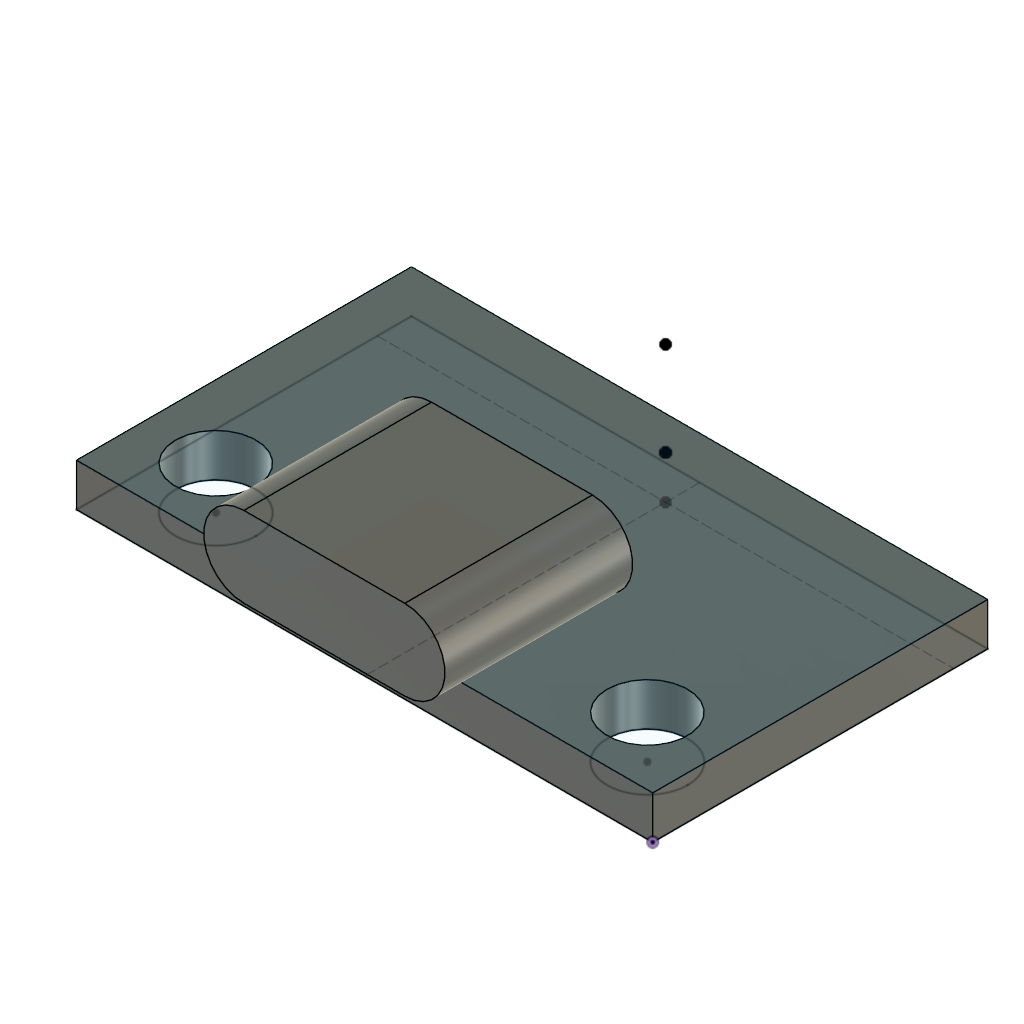
USB-Breakout (Autodesk Fusion 360 design; units mm, degrees)
Autodesk Fusion 360 part; units mm, degrees
sketch "Skizze1" plane through (0, 0, 0) normal (0, 0, 1) x (1, 0, 0)
  line L0 (0, 0) -> (-21.5, 0)
  line L1 (-21.5, 0) -> (-21.5, 12.5)
  line L2 (-21.5, 12.5) -> (0, 12.5)
  line L3 (0, 12.5) -> (0, 0)
  circle A0 centre (-18.8, 2.5) radius 1.5
  circle A1 centre (-2.7, 2.5) radius 1.5
  line L4 (-21.5, 11.23) -> (0, 11.23) construction
  line L5 (-10.75, 12.5) -> (-10.75, 0) construction
  point P0 (-10.75, 11.23)
  dimension "d1" = 21.5
  dimension "d2" = 12.5
  dimension "d3" = 3
  dimension "d4" = 2.7
  dimension "d5" = 2.7
  dimension "d6" = 2.5
  dimension "d7" = 2.5
  dimension "d8" = 1.27
  constraint horizontal L0
  constraint vertical L1
  constraint horizontal L2
  constraint vertical L3
  constraint coincident L0.start L3.end
  constraint equal A0 A1
  constraint coincident L1 L4.start
  constraint coincident L3 L4.end
  constraint perpendicular L3 L4
  constraint midpoint L2 L5.start
  constraint midpoint L0 L5.end
  constraint midpoint L4 P0
  measures "d1" distance of L1.end L2.end
  measures "d2" distance of L0.end L1.end
  measures "d3" diameter of A0
  measures "d4" distance of L1 A0.centre
  measures "d5" distance of L3 A1.centre
  measures "d6" distance of L0 A0.centre
  measures "d7" distance of L0 A1.centre
  measures "d8" distance of L2 L4
extrude "Extrusion1" add sketch "Skizze1" along normal blind 1.6
sketch "Skizze2" plane through (0, 0, 0) normal (0, -1, 0) x (1, 0, 0)
  line L0 (-21.5, 0) -> (0, 0)
  line L1 (0, 0) -> (0, 1.6)
  line L2 (0, 1.6) -> (-21.5, 1.6)
  line L3 (-21.5, 1.6) -> (-21.5, 0)
  line L4 (-10.75, 0) -> (-10.75, 13.6465) construction
  line L5 (-13.75, 4.6) -> (-7.75, 4.6)
  line L6 (-7.75, 1.6) -> (-13.75, 1.6)
  arc A0 (-13.75, 4.6) -> (-13.75, 1.6) centre (-13.75, 3.1) ccw
  arc A1 (-7.75, 1.6) -> (-7.75, 4.6) centre (-7.75, 3.1) ccw
  point P0 (-10.75, 1.6)
  dimension "d11" = 1.5
  dimension "d12" = 6
  constraint midpoint L0 L4.start
  constraint perpendicular L2 L4
  constraint tangent L5 A1
  constraint tangent L6 A0
  constraint tangent L5 A0
  constraint tangent L6 A1
  constraint equal A0 A1
  constraint symmetric L4 L5.start L5.end
  constraint midpoint L2 P0
  constraint coincident L6 P0
  measures "d11" radius of A0
  measures "d12" distance of A0.centre A1.centre
extrude "Extrusion2" add sketch "Skizze2" along normal blind 1.5 and the other way blind 5.5 contours L2 L5 L6 A0 A1
sketch "Skizze3" plane through (0, 0, 1.6) normal (0, 0, 1) x (-1, 0, 0)
  line L0 (7.75, -5.5) -> (7.75, 0)
  line L1 (7.75, 0) -> (0, 0)
  line L2 (0, 0) -> (0, -12.5)
  line L3 (0, -12.5) -> (21.5, -12.5)
  line L4 (21.5, -12.5) -> (21.5, 0)
  line L5 (21.5, 0) -> (13.75, 0)
  line L6 (13.75, 0) -> (13.75, -5.5)
  line L7 (13.75, -5.5) -> (7.75, -5.5)
  circle A0 centre (2.7, -2.5) radius 1.5
  circle A1 centre (18.8, -2.5) radius 1.5
  point P0 (10.75, -11.23)
  point P1 (10.75, -11.23)
  constraint coincident P1 P0
ref_plane "Arbeitsebene1" through (0, 0, 5.1) normal (0, 0, 1) x (1, 0, 0)
sketch "Skizze4" plane through (0, 0, 5.1) normal (0, 0, 1) x (1, 0, 0)
  point P0 (-10.75, 11.23)
  point P1 (-10.75, 11.23)
  constraint coincident P0 P1
equation "d4 = 1.2 mm + 1.5 mm"
equation "d5 = d4"
equation "d7 = d6"
equation "d8 = ( 2.54 / 2 ) * 1 mm"
equation "d12 = 9 mm - 3 mm"
equation "d15 = 7 mm - 1.5 mm"
equation "d17 = 1.6 mm + 3.5 mm"
